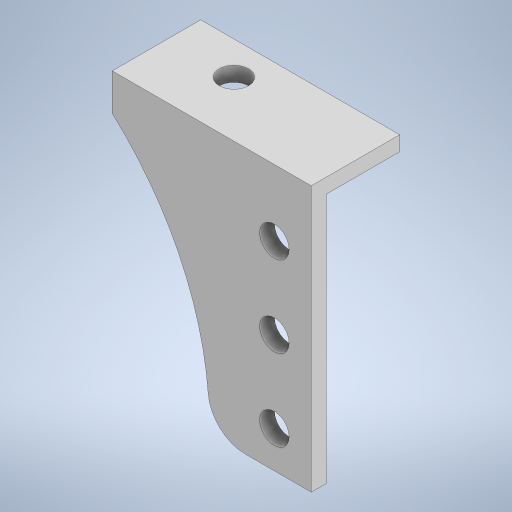
# Autodesk Inventor part: pieza 1-19
Saved by Autodesk Inventor 2024.2 (Build 282272000, 272)
## iProperties
Created: 2024-10-10
Part Number: pieza 1-19
Material: Generic
Document SubType Name: Modeling
Designer: Precisión-18
Density: 1 g/cm^3
Appearance: Default
Author: Precisión-18
Autodesk Inventor part; units mm, degrees
ref_plane "YZ Plane" through (0, 0, 0) normal (1, 0, 0) x (0, 1, 0)
ref_plane "XZ Plane" through (0, 0, 0) normal (0, 1, 0) x (-1, 0, 0)
ref_plane "XY Plane" through (0, 0, 0) normal (0, 0, 1) x (1, 0, 0)
sketch "Sketch1" plane through (0, 0, 0) normal (1, 0, 0) x (0, 1, 0)
  line L0 (0, 0) -> (36, 0)
  line L1 (36, 0) -> (36, -12)
  line L2 (36, -12) -> (34, -12)
  line L3 (34, -12) -> (34, -2)
  line L4 (34, -2) -> (0, -2)
  line L5 (0, -2) -> (0, 0)
  dimension "d0" = 36
  dimension "d1" = 12
  dimension "d2" = 2
  dimension "d3" = 2
  constraints: 12 end point, 3 perpendicular, 2 horizontal, 1 parallel
  measures "d0" distance of L0.start L0.end
  measures "d1" distance of L0.end L1.end
  measures "d2" distance of L1.end L2.end
  measures "d3" distance between parallel lines of L0 L4
extrude "Extrusion1" add sketch "Sketch1" against normal blind 27
sketch "Sketch2" plane through (0, 36, 0) normal (0, 1, 0) x (1, 0, 0)
  circle A0 centre (-18, 7.5) radius 2
  line L0 (0, 0) -> (-27, 0) projected
  line L1 (0, 12) -> (0, 0) projected
  dimension "d6" = 4
  dimension "d7" = 7.5
  dimension "d8" = 18
  constraints: 1 centre point
  measures "d6" diameter of A0
  measures "d7" distance from line of L0 A0.centre
  measures "d8" distance from line of L1 A0.centre
extrude "Extrusion2" cut sketch "Sketch2" against normal blind 27
sketch "Sketch3" plane through (0, 0, 0) normal (0, 0, 1) x (1, 0, 0)
  line L0 (-27, 34) -> (-27, 0) projected
  line L1 (0, 36) -> (-27, 36) projected
  line L2 (-25.8683, 31) -> (-28.3872, 31) construction
  arc A0 (-13.9835, 4.5947) -> (-9, 0) centre (-9, 5) ccw
  line L3 (0, 0) -> (-27, 0) projected
  line L4 (0, 36) -> (0, 0) projected
  line L5 (-14, 4.4018) -> (-14, 0) construction
  circle A1 centre (-5, 27) radius 2
  circle A2 centre (-5, 16) radius 2
  circle A3 centre (-5, 5) radius 2
  line L6 (-27, 36) -> (0, 36)
  line L7 (0, 36) -> (0, 0)
  line L8 (0, 0) -> (-27, 0)
  line L9 (-27, 0) -> (-27, 36)
  arc A4 (-13.9835, 4.5947) -> (-27, 31) centre (-53.8519, 1.3525) ccw
  point P0 (-9, 0)
  dimension "d12" = 5
  dimension "d13" = 10
  dimension "d15" = 4
  dimension "d16" = 4
  dimension "d17" = 4
  dimension "d18" = 5
  dimension "d19" = 16
  dimension "d20" = 27
  dimension "d21" = 5
  dimension "d22" = 5
  dimension "d23" = 5
  dimension "d26" = 14
  dimension "d27" = 40
  constraints: 12 end point, 5 centre point, 4 point on circle, 4 point on line, 3 tangent, 2 horizontal, 2 parallel, 2 perpendicular
  measures "d12" distance from line of L1 A4.end
  measures "d13" diameter of A0
  measures "d15" diameter of A1
  measures "d16" diameter of A2
  measures "d17" diameter of A3
  measures "d18" distance from line of A3.centre L3
  measures "d19" distance from line of L3 A2.centre
  measures "d20" distance from line of L3 A1.centre
  measures "d21" distance from line of L4 A1.centre
  measures "d22" distance from line of L4 A2.centre
  measures "d23" distance from line of L4 A3.centre
  measures "d26" distance between parallel lines of L4 L5
  measures "d27" radius of A4
extrude "Extrusion3" cut sketch "Sketch3" against normal blind 27 contours A4 A0 L3 L0 | A1 | A2 | A3
body "Solid1"
